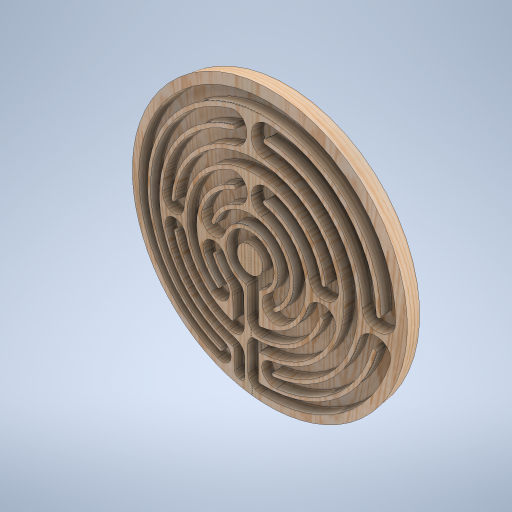
# Autodesk Inventor part: Labiorintas 2
Saved by Autodesk Inventor 2024 (Build 280153000, 153)
## iProperties
Created: 2023-12-19
Part Number: Labiorintas 2
Material: PLW
Document SubType Name: Modeling
Designer: SauliusD
Density: 0.8 g/cm^3
Appearance: PLW
Mass: 426.71 g
Surface Area: 2811.38 cm^2
Volume: 533.387 cm^3
Author: SauliusD
Autodesk Inventor part; units mm, degrees
ref_plane "YZ Plane" through (0, 0, 0) normal (1, 0, 0) x (0, 1, 0)
ref_plane "XZ Plane" through (0, 0, 0) normal (0, 1, 0) x (-1, 0, 0)
ref_plane "XY Plane" through (0, 0, 0) normal (0, 0, 1) x (1, 0, 0)
sketch "Sketch1" plane through (0, 0, 0) normal (0, 0, 1) x (1, 0, 0)
  circle A0 centre (0, 0) radius 160.5
  dimension "d0" = 321
  constraints: 1 centre point, 1 coincident
  measures "d0" diameter of A0
extrude "Extrusion1" add sketch "Sketch1" along normal blind 15
sketch "Sketch2" plane through (0, 0, 15) normal (0, 0, 1) x (1, 0, 0)
  circle A0 centre (0, 0) radius 160.5 projected
  circle A1 centre (0, 0) radius 150.5
  circle A2 centre (0, 0) radius 137.5
  circle A3 centre (0, 0) radius 133.1
  circle A4 centre (0, 0) radius 120.1
  circle A5 centre (0, 0) radius 115.7
  circle A6 centre (0, 0) radius 102.7
  circle A7 centre (0, 0) radius 98.3
  circle A8 centre (0, 0) radius 85.3
  circle A9 centre (0, 0) radius 80.9
  circle A10 centre (0, 0) radius 67.9
  circle A11 centre (0, 0) radius 63.5
  circle A12 centre (0, 0) radius 50.5
  circle A13 centre (0, 0) radius 46.1
  circle A14 centre (0, 0) radius 33.1
  circle A15 centre (0, 0) radius 28.7
  circle A16 centre (0, 0) radius 15.7
  dimension "d3" = 10
  dimension "d4" = 13
  dimension "d5" = 4.4
  dimension "d6" = 13
  dimension "d7" = 4.4
  dimension "d8" = 13
  dimension "d9" = 4.4
  dimension "d10" = 13
  dimension "d11" = 4.4
  dimension "d12" = 13
  dimension "d13" = 4.4
  dimension "d14" = 13
  dimension "d15" = 4.4
  dimension "d16" = 13
  dimension "d17" = 4.4
  dimension "d18" = 13
  constraints: 16 centre point
  measures "d3" radial gap between concentric circles of A0 A1
  measures "d4" radial gap between concentric circles of A1 A2
  measures "d5" radial gap between concentric circles of A2 A3
  measures "d6" radial gap between concentric circles of A3 A4
  measures "d7" radial gap between concentric circles of A4 A5
  measures "d8" radial gap between concentric circles of A5 A6
  measures "d9" radial gap between concentric circles of A6 A7
  measures "d10" radial gap between concentric circles of A7 A8
  measures "d11" radial gap between concentric circles of A8 A9
  measures "d12" radial gap between concentric circles of A9 A10
  measures "d13" radial gap between concentric circles of A10 A11
  measures "d14" radial gap between concentric circles of A11 A12
  measures "d15" radial gap between concentric circles of A12 A13
  measures "d16" radial gap between concentric circles of A13 A14
  measures "d17" radial gap between concentric circles of A14 A15
  measures "d18" radial gap between concentric circles of A15 A16
extrude "Extrusion2" cut sketch "Sketch2" against normal blind 13 contours A1 | A3 | A5 | A7 | A9 | A11 | A13 | A15
sketch "Sketch3" plane through (0, 0, 15) normal (0, 0, 1) x (1, 0, 0)
  line L0 (-80.8701, 2.2) -> (-115.7, 2.2)
  line L1 (-115.7, 2.2) -> (-115.7, -2.2)
  line L2 (-115.7, -2.2) -> (-80.8701, -2.2)
  line L3 (-80.8701, -2.2) -> (-80.8701, 2.2)
  circle A0 centre (0, 0) radius 115.7 projected
  circle A1 centre (0, 0) radius 80.9 projected
  line L4 (-115.7, 2.2) -> (-83.9348, 2.2)
  line L5 (-83.9348, 2.2) -> (-83.9348, 15.2)
  line L6 (-83.9348, 15.2) -> (-115.7, 15.2)
  line L7 (-115.7, 15.2) -> (-115.7, 2.2)
  circle A2 centre (0, 0) radius 85.3 projected
  circle A3 centre (0, 0) radius 160.5 projected
  circle A4 centre (0, 0) radius 133.1 projected
  line L8 (150.5, 2.2) -> (120.0798, 2.2)
  line L9 (120.0798, 2.2) -> (120.0798, -2.2)
  line L10 (120.0798, -2.2) -> (150.5, -2.2)
  line L11 (150.5, -2.2) -> (150.5, 2.2)
  circle A5 centre (0, 0) radius 120.1 projected
  circle A6 centre (0, 0) radius 150.5 projected
  line L12 (119.1343, 2.2) -> (150.5, 2.2)
  line L13 (150.5, 2.2) -> (150.5, 15.2)
  line L14 (150.5, 15.2) -> (119.1343, 15.2)
  line L15 (119.1343, 15.2) -> (119.1343, 2.2)
  line L16 (-28.7, 2.2) -> (-67.8643, 2.2)
  line L17 (-67.8643, 2.2) -> (-67.8643, -2.2)
  line L18 (-67.8643, -2.2) -> (-28.7, -2.2)
  line L19 (-28.7, -2.2) -> (-28.7, 2.2)
  circle A7 centre (0, 0) radius 67.9 projected
  circle A8 centre (0, 0) radius 28.7 projected
  line L20 (-63.5, 15.2) -> (-29.4036, 15.2)
  line L21 (-29.4036, 15.2) -> (-29.4036, 2.2)
  line L22 (-29.4036, 2.2) -> (-63.5, 2.2)
  line L23 (-63.5, 2.2) -> (-63.5, 15.2)
  circle A9 centre (0, 0) radius 63.5 projected
  circle A10 centre (0, 0) radius 33.1 projected
  point P0 (-80.8701, 0)
  point P1 (-115.6791, 2.2)
  point P2 (-115.6791, -2.2)
  point P3 (-85.2716, 2.2)
  point P4 (-114.6972, 15.2)
  point P5 (120.0798, 0)
  point P6 (150.4839, -2.2)
  point P7 (150.4839, 2.2)
  point P8 (149.7305, 15.2)
  point P9 (-28.7, 0)
  point P10 (-33.0268, 2.2)
  point P11 (-61.654, 15.2)
  point P12 (-63.4619, 2.2)
  dimension "d21" = 4.4
  dimension "d24" = 13
  constraints: 48 end point, 12 parallel, 6 collinear, 6 horizontal, 6 perpendicular, 5 tangent, 3 horizontal alignment, 3 midpoint, 2 point on circle, 8 other
  measures "d21" distance of L2.end L0.start
  measures "d24" distance of L4.end L5.end
extrude "Extrusion3" add sketch "Sketch3" against normal up to surface (13 mm away) contours A1 L2 A2 L0 | A2 L2 A0 L0
extrude "Extrusion4" cut sketch "Sketch3" against normal up to surface (13 mm away) contours L0 A0 L6 A2
fillet "Fillet1" radius 15.2 2 edges at (-115.6791, 2.2, 8.5) (-85.2716, 2.2, 8.5)
fillet "Fillet2" radius 2.2 2 edges at (-101.5689, 15.2, 8.5) (-97.1177, 15.2, 8.5)
mirror "Mirror1" about plane through (0, 0, 0) normal (0, 1, 0) of "Extrusion4"
fillet "Fillet3" radius 15.2 2 edges at (-115.6791, -2.2, 8.5) (-85.2716, -2.2, 8.5)
fillet "Fillet4" radius 2.2 2 edges at (-101.5689, -15.2, 8.5) (-97.1177, -15.2, 8.5)
mirror "Mirror2" [suppressed]
fillet "Fillet5" [suppressed]
fillet "Fillet6" [suppressed]
sketch "Sketch8" plane through (0, 0, 15) normal (0, 0, 1) x (1, 0, 0)
  line L0 (67.8643, 2.2) -> (102.6764, 2.2)
  line L1 (102.6764, 2.2) -> (102.6764, -2.2)
  line L2 (102.6764, -2.2) -> (67.8643, -2.2)
  line L3 (67.8643, -2.2) -> (67.8643, 2.2)
  circle A0 centre (0, 0) radius 67.9 projected
  arc A1 (-101.149, -17.7809) -> (-101.149, 17.7809) centre (0, 0) ccw projected
  line L4 (79.4592, 2.2) -> (85.3, 2.2)
  line L5 (85.3, 2.2) -> (85.3, 15.2)
  line L6 (85.3, 15.2) -> (79.4592, 15.2)
  line L7 (79.4592, 15.2) -> (79.4592, 2.2)
  line L8 (79.4592, -2.2) -> (85.3, -2.2)
  line L9 (85.3, -2.2) -> (85.3, -15.2)
  line L10 (85.3, -15.2) -> (79.4592, -15.2)
  line L11 (79.4592, -15.2) -> (79.4592, -2.2)
  circle A2 centre (0, 0) radius 80.9 projected
  arc A3 (-84.0118, -14.7684) -> (-84.0118, 14.7684) centre (0, 0) ccw projected
  point P0 (67.8643, 0)
  dimension "d86" = 4.4
  dimension "d87" = 13
  constraints: 24 end point, 6 parallel, 4 point on line, 3 horizontal, 3 perpendicular, 1 collinear, 1 horizontal alignment, 1 midpoint, 1 point on circle, 1 tangent, 4 other
  measures "d86" distance of L2.end L0.start
  measures "d87" distance of L6.end L4.start
extrude "Extrusion15" add sketch "Sketch8" against normal up to surface (13 mm away) contours A0 L3 | L0 A2 L2 A0 | L0 A3 L2 A2 | L0 L1 L2 A3 picked at (67.8709, -0.4889)
extrude "Extrusion16" cut sketch "Sketch8" against normal up to surface (13 mm away) contours L7 A2 L0 | A2 L6 A3 L0 | L2 A2 L11 | A3 L6 L5 L0 | A2 L2 A3 L10 | L2 L9 L10 A3
extrude "Extrusion6" add sketch "Sketch3" against normal up to surface (13 mm away) contours A4 L10 A5 L8 | A4 L8 A6 L10
extrude "Extrusion7" cut sketch "Sketch3" against normal up to surface (13 mm away) contours L8 A5 L14 A4 | A4 L14 A6 L8
mirror "Mirror3" about plane through (0, 0, 0) normal (0, 1, 0) of "Extrusion7"
fillet "Fillet7" radius 15.2 4 edges at (120.0798, 2.2, 8.5) (150.4839, 2.2, 8.5) (120.0798, -2.2, 8.5) (150.4839, -2.2, 8.5)
fillet "Fillet8" radius 2.2 4 edges at (132.2292, 15.2, 8.5) (136.6573, 15.2, 8.5) (132.2292, -15.2, 8.5) (136.6573, -15.2, 8.5)
extrude "Extrusion8" add sketch "Sketch3" against normal up to surface (13 mm away) contours L19 L18 A10 L16 | A10 L18 A9 L16 | A9 L18 L17 L16
extrude "Extrusion9" cut sketch "Sketch3" against normal up to surface (13 mm away) contours L16 A9 L20 A10
mirror "Mirror4" about plane through (0, 0, 0) normal (0, 1, 0) of "Extrusion9"
fillet "Fillet9" radius 15.2 4 edges at (-63.4619, -2.2, 8.5) (-33.0268, -2.2, 8.5) (-63.4619, 2.2, 8.5) (-33.0268, 2.2, 8.5)
fillet "Fillet10" radius 2.2 4 edges at (-48.1582, 15.2, 8.5) (-43.5221, 15.2, 8.5) (-48.1582, -15.2, 8.5) (-43.5221, -15.2, 8.5)
sketch "Paveiksliukas" plane through (0, 0, 15) normal (0, 0, 1) x (1, 0, 0)
  line L0 (-160.3373, 159.9944) -> (160.6852, 159.9944) construction
  line L1 (160.6852, 159.9944) -> (160.6852, -160.5388) construction
  line L2 (160.6852, -160.5388) -> (-160.3373, -160.5388) construction
  line L3 (-160.3373, -160.5388) -> (-160.3373, 159.9944) construction
  point P0 (0, 0)
  constraints: 2 other
sketch "Sketch5" plane through (0, 0, 15) normal (0, 0, 1) x (1, 0, 0)
  line L0 (2.2, 137.4824) -> (-2.2, 137.4824)
  line L1 (-2.2, 137.4824) -> (-2.2, 98.2754)
  line L2 (-2.2, 98.2754) -> (2.2, 98.2754)
  line L3 (2.2, 98.2754) -> (2.2, 137.4824)
  line L4 (2.2, 85.2716) -> (-2.2, 85.2716)
  line L5 (-2.2, 85.2716) -> (-2.2, 46.0475)
  line L6 (-2.2, 46.0475) -> (2.2, 46.0475)
  line L7 (2.2, 46.0475) -> (2.2, 85.2716)
  arc A0 (136.3582, 17.6829) -> (136.3582, -17.6829) centre (0, 0) ccw projected
  arc A1 (-84.0118, -14.7684) -> (-84.0118, 14.7684) centre (0, 0) ccw projected
  arc A2 (-43.0047, -16.6075) -> (-43.0047, 16.6075) centre (0, 0) ccw projected
  arc A3 (-96.8155, -17.0191) -> (-96.8155, 17.0191) centre (0, 0) ccw projected
  line L8 (15.2, 136.6573) -> (2.2, 136.6573)
  line L9 (2.2, 136.6573) -> (2.2, 98.2754)
  line L10 (2.2, 98.2754) -> (15.2, 98.2754)
  line L11 (15.2, 98.2754) -> (15.2, 136.6573)
  arc A4 (-101.149, -17.7809) -> (-101.149, 17.7809) centre (0, 0) ccw projected
  arc A5 (131.9948, 17.1171) -> (131.9948, -17.1171) centre (0, 0) ccw projected
  line L12 (2.2, 83.9348) -> (15.2, 83.9348)
  line L13 (15.2, 83.9348) -> (15.2, 46.0475)
  line L14 (15.2, 46.0475) -> (2.2, 46.0475)
  line L15 (2.2, 46.0475) -> (2.2, 83.9348)
  arc A6 (79.4592, 15.2) -> (79.4592, -15.2) centre (0, 0) ccw projected
  arc A7 (-47.1092, -18.1925) -> (-47.1092, 18.1925) centre (0, 0) ccw projected
  point P0 (0, 46.0475)
  point P1 (0, 98.2754)
  point P2 (84.0364, 14.6277)
  point P3 (96.8155, 17.0191)
  point P4 (101.149, 17.7809)
  point P5 (2.2, 50.4521)
  point P6 (15.2, 48.1582)
  point P7 (15.2, 79.4592)
  point P8 (2.2, 80.8701)
  point P9 (15.2, 132.2292)
  point P10 (2.2, 133.0818)
  point P11 (2.2, 102.6764)
  point P12 (15.2, 101.5689)
  dimension "d63" = 4.4
  dimension "d64" = 13
  constraints: 32 end point, 8 parallel, 8 point on circle, 4 horizontal, 4 perpendicular, 3 collinear, 2 midpoint, 2 point on line, 2 vertical alignment
  measures "d63" distance of L0.start L0.end
  measures "d64" distance of L8.start L8.end
extrude "Extrusion10" add sketch "Sketch5" against normal up to surface (13 mm away) contours L3 A5 L1 L0 | A5 L3 A4 L1 | A4 L3 A3 L1 | A3 L2 | L7 A6 L5 L4 | A6 L7 A7 L5 | A7 L7 A2 L5 | A2 L6
extrude "Extrusion11" cut sketch "Sketch5" against normal up to surface (13 mm away) contours A5 L11 A4 L3 | A6 L13 A7 L7
mirror "Mirror5" about plane through (0, 0, 0) normal (1, 0, 0) of "Extrusion11"
fillet "Fillet11" radius 15.2 4 edges at (-2.2, 102.6764, 8.5) (-2.2, 133.0818, 8.5) (2.2, 133.0818, 8.5) (2.2, 102.6764, 8.5)
fillet "Fillet12" radius 15 4 edges at (2.2, 80.8701, 8.5) (2.2, 50.4521, 8.5) (-2.2, 80.8701, 8.5) (-2.2, 50.4521, 8.5)
fillet "Fillet13" radius 2.2 8 edges at (15.2, 119.1343, 8.5) (15.2, 114.6972, 8.5) (15.2, 66.1768, 8.5) (15.2, 61.654, 8.5) (-15.2, 66.1768, 8.5) (-15.2, 61.654, 8.5) (-15.2, 119.1343, 8.5) (-15.2, 114.6972, 8.5)
sketch "Sketch6" plane through (0, 0, 15) normal (0, 0, 1) x (1, 0, 0)
  line L0 (-22, -117.1625) -> (-26.4, -117.1625)
  line L1 (-26.4, -117.1625) -> (-26.4, -148.8833)
  line L2 (-26.4, -148.8833) -> (-22, -148.8833)
  line L3 (-22, -148.8833) -> (-22, -117.1625)
  line L4 (-22, -40.5119) -> (-26.4, -40.5119)
  line L5 (-26.4, -40.5119) -> (-26.4, -81.1118)
  line L6 (-26.4, -81.1118) -> (-22, -81.1118)
  line L7 (-22, -81.1118) -> (-22, -40.5119)
  arc A0 (149.2503, 19.3548) -> (149.2503, -19.3548) centre (0, 0) ccw projected
  arc A1 (-17.7247, 118.7849) -> (119.1027, -15.4452) centre (0, 0) ccw projected
  arc A2 (-84.0118, -14.7684) -> (-84.0118, 14.7684) centre (0, 0) ccw projected
  arc A3 (-43.0047, -16.6075) -> (2.2, 46.0475) centre (0, 0) ccw projected
  line L8 (-3.3, -28.5096) -> (-7.7, -28.5096)
  line L9 (-7.7, -28.5096) -> (-7.7, -150.4638)
  line L10 (-7.7, -150.4638) -> (-3.3, -150.4638)
  line L11 (-3.3, -150.4638) -> (-3.3, -28.5096)
  circle A4 centre (0, 0) radius 28.7 projected
  line L12 (-26.4, -43.0499) -> (-39.4, -43.0499)
  line L13 (-39.4, -43.0499) -> (-39.4, -70.6573)
  line L14 (-39.4, -70.6573) -> (-26.4, -70.6573)
  line L15 (-26.4, -70.6573) -> (-26.4, -43.0499)
  arc A5 (-47.1092, -18.1925) -> (13.2611, 48.7278) centre (0, 0) ccw projected
  arc A6 (-21.115, 78.0959) -> (21.115, 78.0959) centre (0, 0) ccw projected
  line L16 (-26.4, -117.1625) -> (-39.4, -117.1625)
  line L17 (-39.4, -117.1625) -> (-39.4, -145.2511)
  line L18 (-39.4, -145.2511) -> (-26.4, -145.2511)
  line L19 (-26.4, -145.2511) -> (-26.4, -117.1625)
  line L20 (-7.7, -102.4109) -> (-22, -102.4109)
  line L21 (-22, -102.4109) -> (-22, -150.3029)
  line L22 (-22, -150.3029) -> (-7.7, -150.3029)
  line L23 (-7.7, -150.3029) -> (-7.7, -102.4109)
  arc A7 (-101.149, -17.7809) -> (15.1567, 101.5754) centre (0, 0) ccw projected
  line L24 (-3.3, -85.2361) -> (10.6204, -85.2361)
  line L25 (10.6204, -85.2361) -> (10.6204, -150.1248)
  line L26 (10.6204, -150.1248) -> (-3.3, -150.1248)
  line L27 (-3.3, -150.1248) -> (-3.3, -85.2361)
  line L28 (10.6204, -26.6626) -> (-3.3, -26.6626)
  line L29 (-3.3, -26.6626) -> (-3.3, -80.1999)
  line L30 (-3.3, -80.1999) -> (10.6204, -80.1999)
  line L31 (10.6204, -80.1999) -> (10.6204, -26.6626)
  line L32 (10.6204, -101.5957) -> (15.0204, -101.5957)
  line L33 (15.0204, -101.5957) -> (15.0204, -136.6771)
  line L34 (15.0204, -136.6771) -> (10.6204, -136.6771)
  line L35 (10.6204, -136.6771) -> (10.6204, -101.5957)
  arc A8 (136.3582, 17.6829) -> (136.3582, -17.6829) centre (0, 0) ccw projected
  line L36 (10.6204, -26.6626) -> (15.0204, -26.6626)
  line L37 (15.0204, -26.6626) -> (15.0204, -66.2178)
  line L38 (15.0204, -66.2178) -> (10.6204, -66.2178)
  line L39 (10.6204, -66.2178) -> (10.6204, -26.6626)
  arc A9 (-17.9826, 65.4754) -> (17.9826, 65.4754) centre (0, 0) ccw projected
  line L40 (-7.7, -32.1919) -> (-22, -32.1919)
  line L41 (-22, -32.1919) -> (-22, -95.8065)
  line L42 (-22, -95.8065) -> (-7.7, -95.8065)
  line L43 (-7.7, -95.8065) -> (-7.7, -32.1919)
  arc A10 (-30.8775, -11.9242) -> (-30.8775, 11.9242) centre (0, 0) ccw projected
  arc A11 (-2.2, 98.2754) -> (-96.8155, 17.0191) centre (0, 0) ccw projected
  point P0 (84.0364, -14.6277)
  point P1 (101.149, -17.7809)
  point P2 (-22, -118.0678)
  point P3 (-26.4, -148.1664)
  point P4 (-3.3, -150.1248)
  point P5 (-7.7, -150.3029)
  point P6 (-22, -77.8512)
  point P7 (96.8155, -17.0191)
  point P8 (-96.8155, -17.0191)
  dimension "d72" = 4.4
  dimension "d73" = 22
  dimension "d74" = 3.3
  dimension "d75" = 4.4
  dimension "d76" = 13
  dimension "d77" = 13.9204
  dimension "d78" = 4.4
  constraints: 88 end point, 22 parallel, 21 point on circle, 11 collinear, 11 horizontal, 11 perpendicular, 3 point on line
  measures "d72" distance of L1.end L2.end
  measures "d73" distance from line of point (0, 0) L3
  measures "d74" distance from line of point (0, 0) L11
  measures "d75" distance of L8.start L8.end
  measures "d76" distance of L12.start L12.end
  measures "d77" distance of L24.start L24.end
  measures "d78" distance of L32.start L32.end
extrude "Extrusion12" add sketch "Sketch6" against normal up to surface (13 mm away) contours A1 L3 A8 L1 | A8 L3 A0 L1 | L9 A7 L11 A1 | A1 L11 A8 L9 | L9 A2 L11 A7 | A8 L11 A0 L9 | A0 L10 L9 | L25 A7 L33 A1 | A1 L33 L34 L25 | L9 A6 L11 A2 | L25 L32 A7 | L9 A9 L11 A6 | L5 A6 L7 L6 | L9 A5 L11 A9 | A6 L5 A9 L7 | L9 A3 L11 A5 | A9 L5 A5 L7 | L9 A10 L11 A3 | A5 L5 L4 L7 | L31 A5 L37 L38 | L9 L8 L11 A10 | L31 A3 L37 A5 | L31 A10 L37 A3 | L31 L36 L37 A10
extrude "Extrusion13" cut sketch "Sketch6" against normal up to surface (13 mm away) contours L21 L20 L9 A1 L3 | L1 A8 L17 L16 | A1 L9 A8 L3 | L1 L18 L17 A8 | A8 L9 A0 L3 | A0 L22 L21 | L11 A7 L25 A1 | A1 L25 A8 L11 | L42 L41 A2 L9 | L11 A2 L24 L25 A7 | A8 L25 L26 L11 | A2 L41 L7 A6 L9 | L24 A2 | A6 L7 A9 L9 | A9 L7 A5 L9 | L11 A9 L31 L30 | A5 L7 A3 L9 | L11 A5 L31 A9 | L14 L13 A9 L5 | A3 L41 L40 L9 | L11 A3 L31 A5 | A9 L13 L12 L5 | L11 A10 L31 A3 | L11 A4 L31 A10 | L29 L28 A4 picked at (4.4746, -27.1229)
sketch "Sketch7" plane through (0, 0, 15) normal (0, 0, 1) x (1, 0, 0)
  line L0 (15.0204, -29.4957) -> (15.0204, -43.5844) projected
  arc A0 (15.0204, -61.698) -> (16.8174, 61.2326) centre (0, 0) ccw projected
  line L1 (15.0204, -29.4957) -> (28.0204, -29.4957)
  line L2 (28.0204, -29.4957) -> (28.0204, -56.9834)
  line L3 (28.0204, -56.9834) -> (15.0204, -56.9834)
  line L4 (15.0204, -56.9834) -> (15.0204, -29.4957)
  line L5 (28.0204, -101.5957) -> (15.0204, -101.5957)
  line L6 (15.0204, -101.5957) -> (15.0204, -130.1171)
  line L7 (15.0204, -130.1171) -> (28.0204, -130.1171)
  line L8 (28.0204, -130.1171) -> (28.0204, -101.5957)
  line L9 (15.0204, -114.7209) -> (15.0204, -101.5957) projected
  arc A1 (15.0204, -132.2498) -> (131.9948, -17.1171) centre (0, 0) ccw projected
  arc A2 (-101.149, -17.7809) -> (-7.7, -102.4109) centre (0, 0) ccw projected
  point P0 (101.149, -17.7809)
  dimension "d83" = 13
  constraints: 16 end point, 4 parallel, 3 point on circle, 2 collinear, 2 horizontal, 2 perpendicular
  measures "d83" distance of L0.start L1.end
extrude "Extrusion14" cut sketch "Sketch7" against normal up to surface (13 mm away)
fillet "Fillet17" radius 2.2 12 edges at (-39.4, -131.7342, 8.5) (-39.4, -127.1348, 8.5) (-39.4, -55.2996, 8.5) (-39.4, -49.7985, 8.5) (28.0204, -42.0132, 8.5) (28.0204, -36.6069, 8.5) (79.4592, -15.2, 8.5) (83.9348, -15.2, 8.5) (79.4592, 15.2, 8.5) (83.9348, 15.2, 8.5) (28.0204, -116.7856, 8.5) (28.0204, -112.2557, 8.5)
fillet "Fillet18" radius 15.2 8 edges at (-26.4, -148.1664, 8.5) (-26.4, -117.1625, 8.5) (-26.4, -76.4712, 8.5) (-26.4, -43.0499, 8.5) (15.0204, -101.5957, 8.5) (15.0204, -132.2498, 8.5) (15.0204, -61.698, 8.5) (15.0204, -29.4957, 8.5)
fillet "Fillet19" radius 19.6 1 edges at (-22, -40.5119, 8.5)
fillet "Fillet21" radius 2.2 7 edges at (-22, -82.4141, 8.5) (-22, -113.5891, 8.5) (-3.3, -28.5096, 8.5) (10.6204, -26.6626, 8.5) (10.6204, -67.0643, 8.5) (10.6204, -137.0892, 8.5) (10.6204, -97.7246, 8.5)
fillet "Fillet22" radius 15.2 6 edges at (-7.7, -32.1919, 8.5) (-7.7, -102.4109, 8.5) (-7.7, -97.998, 8.5) (-3.3, -85.2361, 8.5) (-3.3, -150.4638, 8.5) (-3.3, -80.8327, 8.5)
fillet "Fillet20" radius 6.5 2 edges at (-22, -150.3029, 8.5) (-7.7, -150.3029, 8.5)
fillet "Fillet23" radius 15.2 4 edges at (67.8643, -2.2, 8.5) (98.2754, -2.2, 8.5) (67.8643, 2.2, 8.5) (98.2754, 2.2, 8.5)
equation "\"d4\" = GriovelioS"
equation "\"d5\" = SienelesS"
equation "\"d6\" = GriovelioS"
equation "\"d7\" = SienelesS"
equation "\"d8\" = GriovelioS"
equation "\"d9\" = SienelesS"
equation "\"d10\" = GriovelioS"
equation "\"d11\" = SienelesS"
equation "\"d12\" = GriovelioS"
equation "\"d13\" = SienelesS"
equation "\"d14\" = GriovelioS"
equation "\"d15\" = SienelesS"
equation "\"d16\" = GriovelioS"
equation "\"d17\" = SienelesS"
equation "\"d18\" = GriovelioS"
equation "\"d21\" = SienelesS"
equation "\"d24\" = GriovelioS"
equation "\"d28\" = 0.5 * SienelesS"
equation "\"d30\" = 0.5 * SienelesS"
equation "\"d32\" = 0.5 * SienelesS"
equation "\"d86\" = SienelesS"
equation "\"d87\" = GriovelioS"
equation "\"d40\" = 0.5 * SienelesS"
equation "\"d46\" = 0.5 * SienelesS"
equation "\"d63\" = SienelesS"
equation "\"d64\" = GriovelioS"
equation "\"d71\" = 0.5 * SienelesS"
equation "\"d72\" = SienelesS"
equation "\"d75\" = SienelesS"
equation "\"d76\" = GriovelioS"
equation "\"d78\" = SienelesS"
equation "\"d83\" = GriovelioS"
equation "\"GriovelioS\" = 13"
equation "\"SienelesS\" = 4.4"
body "Solid1"
